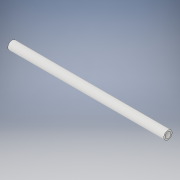
# Autodesk Inventor part: ARM_009_13inSpacerPVC
Saved by Autodesk Inventor 2018.3 (Build 223284000, 284)
## iProperties
Created: 2020-02-01
Part Number: ARM_009_13inSpacerPVC
Material: PVC-Piping
Document SubType Name: Modeling
Designer: 21vogecale
Density: 1.4 g/cm^3
Appearance: Smooth - White
Author: 21vogecale
Autodesk Inventor part; units mm, degrees
ref_plane "YZ Plane" through (0, 0, 0) normal (1, 0, 0) x (0, 1, 0)
ref_plane "XZ Plane" through (0, 0, 0) normal (0, 1, 0) x (-1, 0, 0)
ref_plane "XY Plane" through (0, 0, 0) normal (0, 0, 1) x (1, 0, 0)
sketch "Sketch1" plane through (0, 0, 0) normal (1, 0, 0) x (0, 1, 0)
  circle A0 centre (0, 0) radius 6.35
  circle A1 centre (0, 0) radius 8.89
  dimension "d0" = 12.7
  dimension "d1" = 2.54
  constraints: 2 centre point, 2 coincident
  measures "d0" diameter of A0
  measures "d1" radial gap between concentric circles of A1 A0
extrude "Extrusion1" add sketch "Sketch1" along normal blind 673.1
sketch "Sketch2" plane through (0, 0, 0) normal (0, 1, 0) x (-1, 0, 0)
  line L0 (0, -8.89) -> (0, 8.89) projected
  line L1 (0, -8.89) -> (-330.2, -8.89)
  line L2 (0, -8.89) -> (-673.1, -8.89) projected
  line L3 (-330.2, -8.89) -> (-897.1642, -8.89)
  line L4 (-897.1642, -8.89) -> (-897.1642, 264.8515)
  line L5 (-897.1642, 264.8515) -> (-330.2, 264.8515)
  line L6 (-330.2, 264.8515) -> (-330.2, -8.89)
  point P0 (0, 0)
  dimension "d4" = 330.2
  constraints: 10 end point, 2 parallel, 1 horizontal, 1 perpendicular, 1 point on line
  measures "d4" distance of L0.start L1.end
extrude "Extrusion2" cut sketch "Sketch2" along normal mid plane 25.4
body "Solid1"
